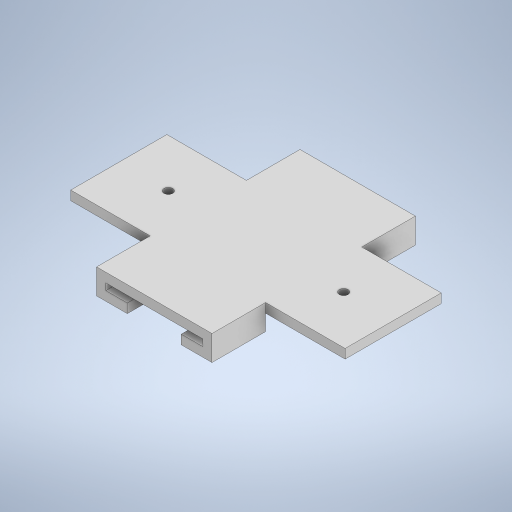
# Autodesk Inventor part: cam_holder
Saved by Autodesk Inventor 2024.3 (Build 283343000, 343)
## iProperties
Created: 2024-12-12
Part Number: cam_holder
Material: Generic
Document SubType Name: Modeling
Designer: User
Density: 1 g/cm^3
Appearance: Default
Author: User
Autodesk Inventor part; units mm, degrees
ref_plane "YZ Plane" through (0, 0, 0) normal (1, 0, 0) x (0, 1, 0)
ref_plane "XZ Plane" through (0, 0, 0) normal (0, 1, 0) x (-1, 0, 0)
ref_plane "XY Plane" through (0, 0, 0) normal (0, 0, 1) x (1, 0, 0)
sketch "Sketch3" plane through (0, 0, 0) normal (0, 1, 0) x (-1, 0, 0)
  line L0 (-74.2, 0) -> (-74.2, -26)
  line L1 (0, -26) -> (0, 0)
  line L2 (0, 0) -> (-24, 0)
  line L3 (-24, 0) -> (-24, 14.5)
  line L4 (-24, 14.5) -> (-50.2, 14.5)
  line L5 (-50.2, 14.5) -> (-50.2, 0)
  line L6 (-50.2, -26) -> (-50.2, -40.5)
  line L7 (-50.2, -40.5) -> (-24, -40.5)
  line L8 (-24, -40.5) -> (-24, -26)
  line L9 (0, -13) -> (-13.4, -13)
  line L10 (-74.2, -13) -> (-60.8, -13)
  line L11 (0, 0) -> (-24, 0)
  line L12 (-50.2, 0) -> (-74.2, 0)
  line L13 (-74.2, -26) -> (-50.2, -26)
  line L14 (-24, -26) -> (0, -26)
  circle A0 centre (-13.4, -13) radius 1.2
  circle A1 centre (-60.8, -13) radius 1.2
  dimension "d2" = 74.2
  dimension "d3" = 26
  dimension "d4" = 24
  dimension "d5" = 14.5
  dimension "d6" = 26.2
  dimension "d7" = 14.5
  dimension "d8" = 26.2
  dimension "d9" = 13.4
  dimension "d10" = 13.4
  dimension "d11" = 2.4
  dimension "d12" = 2.4
  constraints: 30 end point, 9 perpendicular, 5 horizontal, 5 parallel, 2 centre point, 2 coincident, 2 midpoint, 2 point on line
  measures "d2" distance of L1.start L0.end
  measures "d3" distance of L0.end L0.start
  measures "d4" distance of L1.end L2.end
  measures "d5" distance of L2.end L3.end
  measures "d6" distance of L3.end L4.end
  measures "d7" distance of L6.start L6.end
  measures "d8" distance of L6.end L7.end
  measures "d9" distance of L9.start L9.end
  measures "d10" distance of L10.start L10.end
  measures "d11" diameter of A0
  measures "d12" diameter of A1
extrude "Extrusion1" add sketch "Sketch3" along normal blind 2.5
sketch "Sketch4" plane through (50.2, 0, 14.5) normal (1, 0, 0) x (0, 0, -1)
  point P0 (14.5, 0)
sketch "Sketch5" plane through (0, 2.5, 0) normal (0, 1, 0) x (1, 0, 0)
  line L0 (24, -14.5) -> (50.2, -14.5) projected
  line L1 (24, -14.5) -> (21.5, -14.5)
  line L2 (21.5, -14.5) -> (21.5, 0)
  line L3 (21.5, 0) -> (24, 0)
  line L4 (24, 0) -> (24, -14.5)
  point P0 (0, 0)
  dimension "d15" = 2.5
  constraints: 8 end point, 3 perpendicular, 1 horizontal
  measures "d15" distance of L0.start L1.end
extrude "Extrusion2" add sketch "Sketch5" against normal blind 6.8
sketch "Sketch6" plane through (0, 2.5, 0) normal (0, 1, 0) x (1, 0, 0)
  line L0 (50.2, -14.5) -> (50.2, 0) projected
  line L1 (50.2, -14.5) -> (52.7, -14.5)
  line L2 (52.7, -14.5) -> (52.7, 0)
  line L3 (50.2, 0) -> (74.2, 0) projected
  line L4 (50.2, 0) -> (50.2, -14.5)
  point P0 (0, 0)
  dimension "d18" = 2.5
  constraints: 6 end point, 1 horizontal, 1 parallel, 1 perpendicular, 1 point on line
  measures "d18" distance of L0.start L1.end
extrude "Extrusion3" add sketch "Sketch6" against normal blind 6.8
sketch "Sketch7" plane through (0, 2.5, 0) normal (0, 1, 0) x (1, 0, 0)
  line L0 (24, 40.5) -> (24, 26) projected
  line L1 (24, 40.5) -> (21.5, 40.5)
  line L2 (21.5, 40.5) -> (21.5, 26)
  line L3 (21.5, 26) -> (24, 26)
  line L4 (24, 26) -> (24, 40.5)
  point P0 (0, 0)
  dimension "d21" = 2.5
  constraints: 8 end point, 2 perpendicular, 1 collinear, 1 horizontal
  measures "d21" distance of L0.start L1.end
extrude "Extrusion4" add sketch "Sketch7" against normal blind 6.8
sketch "Sketch8" plane through (0, 2.5, 0) normal (0, 1, 0) x (1, 0, 0)
  line L0 (50.2, 26) -> (50.2, 40.5) projected
  line L1 (50.2, 40.5) -> (52.7, 40.5)
  line L2 (52.7, 40.5) -> (52.7, 26)
  line L3 (52.7, 26) -> (50.2, 26)
  line L4 (50.2, 26) -> (50.2, 40.5)
  point P0 (0, 0)
  dimension "d24" = 2.5
  constraints: 8 end point, 2 perpendicular, 1 collinear, 1 horizontal
  measures "d24" distance of L0.end L1.end
extrude "Extrusion5" add sketch "Sketch8" against normal blind 6.8
sketch "Sketch9" plane through (24, 0, -26) normal (1, 0, 0) x (0, 0, -1)
  line L0 (14.5, 0) -> (14.5, -4.3) projected
  line L1 (14.5, -4.3) -> (14.5, -1.8)
  line L2 (14.5, -1.8) -> (0, -1.8)
  line L3 (0, -1.8) -> (0, -4.3)
  line L4 (0, -4.3) -> (14.5, -4.3)
  point P0 (-26, 0)
  dimension "d27" = 2.5
  constraints: 8 end point, 3 perpendicular, 1 point on line
  measures "d27" distance of L0.end L1.end
extrude "Extrusion6" add sketch "Sketch9" along normal blind 5.8
sketch "Sketch10" plane through (50.2, 0, -40.5) normal (-1, 0, 0) x (0, 0, 1)
  line L0 (0, 0) -> (0, -4.3) projected
  line L1 (0, -4.3) -> (0, -1.8)
  line L2 (0, -1.8) -> (14.5, -1.8)
  line L3 (14.5, 0) -> (14.5, -4.3) projected
  line L4 (14.5, -1.8) -> (14.5, -4.3)
  line L5 (14.5, -4.3) -> (0, -4.3)
  point P0 (40.5, 0)
  dimension "d30" = 2.5
  constraints: 8 end point, 2 perpendicular, 1 horizontal, 1 point on line
  measures "d30" distance of L0.end L1.end
extrude "Extrusion7" add sketch "Sketch10" along normal blind 5.8
sketch "Sketch11" plane through (50.2, 0, 0) normal (-1, 0, 0) x (0, 0, 1)
  line L0 (14.5, -4.3) -> (0, -4.3) projected
  line L1 (0, -4.3) -> (0, -1.8)
  line L2 (0, 0) -> (0, -4.3) projected
  arc A0 (-2.0781, -1.1028) -> (0, -1.8) centre (0, 1.6455) ccw
  line L3 (0, -1.8) -> (14.5, -1.8)
  line L4 (14.5, -1.8) -> (14.5, -4.3)
  line L5 (0, 0) -> (0, -4.3) projected
  line L6 (14.5, 2.5) -> (14.5, -4.3) projected
  line L7 (0, -4.3) -> (14.5, -4.3)
  dimension "d33" = 2.5
  constraints: 8 end point, 2 point on circle, 2 point on line, 1 centre point, 1 horizontal, 1 parallel, 1 perpendicular
  measures "d33" distance of L0.end L1.end
extrude "Extrusion8" add sketch "Sketch11" along normal blind 5.8
sketch "Sketch12" plane through (24, 0, 14.5) normal (1, 0, 0) x (0, 0, -1)
  line L0 (0, 0) -> (0, -4.3) projected
  line L1 (0, -4.3) -> (0, -1.8)
  line L2 (0, -1.8) -> (14.5, -1.8)
  line L3 (14.5, -4.3) -> (0, -4.3) projected
  line L4 (14.5, -1.8) -> (14.5, -4.3)
  line L5 (14.5, -4.3) -> (0, -4.3)
  point P0 (14.5, 0)
  dimension "d36" = 2.5
  constraints: 8 end point, 2 perpendicular, 1 collinear, 1 point on line
  measures "d36" distance of L0.end L1.end
extrude "Extrusion9" add sketch "Sketch12" along normal blind 5.8
body "Solid1"
